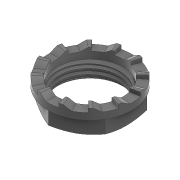
# Autodesk Inventor part: Switch Nut
Saved by Autodesk Inventor 2020 (Build 240168000, 168)
## iProperties
Created: 2019-11-13
Part Number: Switch Nut
Material: Generic
Document SubType Name: Modeling
Designer: amsmi
Density: 1 g/cm^3
Appearance: Default
Author: amsmi
Autodesk Inventor part; units mm, degrees
ref_plane "YZ Plane" through (0, 0, 0) normal (1, 0, 0) x (0, 1, 0)
ref_plane "XZ Plane" through (0, 0, 0) normal (0, 1, 0) x (-1, 0, 0)
sketch "Sketch1" plane through (0, 0, 0) normal (0, 1, 0) x (-1, 0, 0)
  circle A0 centre (0, 0) radius 5.842
  line L0 (6.985, 4.0328) -> (6.985, -4.0328)
  line L1 (6.985, -4.0328) -> (0, -8.0656)
  line L2 (0, -8.0656) -> (-6.985, -4.0328)
  line L3 (-6.985, -4.0328) -> (-6.985, 4.0328)
  line L4 (-6.985, 4.0328) -> (0, 8.0656)
  line L5 (0, 8.0656) -> (6.985, 4.0328)
  dimension "d0" = 11.684
  dimension "d1" = 13.97
  constraints: 12 end point, 2 coincident, 1 centre point, 1 vertical, 13 other
  measures "d0" diameter of A0
  measures "d1" distance between parallel lines of L3 L0
extrude "Extrusion1" add sketch "Sketch1" along normal blind 3.175
sketch "Sketch2" plane through (0, 3.175, 0) normal (0, 1, 0) x (1, 0, 0)
  circle A0 centre (0, 0) radius 8.128
  circle A1 centre (0, 0) radius 6.35
  dimension "d4" = 16.256
  dimension "d5" = 12.7
  constraints: 2 centre point, 2 coincident
  measures "d4" diameter of A0
  measures "d5" diameter of A1
extrude "Extrusion2" add sketch "Sketch2" along normal blind 2.159
chamfer "Chamfer1" distance 0.508 angle 45 2 edges at (5.842, 3.175, 0) (5.842, 0, 0)
sketch "Sketch3" plane through (0, 0, 0) normal (0, -1, 0) x (1, 0, 0)
  circle A0 centre (0, 0) radius 6.985
  line L0 (6.985, -4.0328) -> (0, -8.0656) projected
  constraints: 1 centre point, 1 coincident, 1 tangent
extrude "Extrusion3" cut sketch "Sketch3" against normal through all draft 60 keep common part
sketch "Sketch4" plane through (0, 0, 0) normal (0, 0, 1) x (1, 0, 0)
  line L0 (-1.905, 5.334) -> (-1.905, 4.445) construction
  line L1 (-1.905, 4.445) -> (0.381, 4.445) construction
  line L2 (0.381, 4.445) -> (1.905, 5.334) construction
  line L3 (1.905, 5.334) -> (-1.905, 5.334) construction
  line L4 (-6.35, 5.334) -> (6.35, 5.334) construction
  point P0 (0, 0)
  point P1 (0, 5.334)
  point P2 (0, 4.8895)
  point P3 (1.143, 4.8895)
  dimension "d29" = 3.81
  dimension "d30" = 2.286
  dimension "d31" = 0.889
  constraints: 8 end point, 2 horizontal, 2 midpoint, 2 vertical alignment, 1 horizontal alignment, 1 point on line, 1 vertical
  measures "d29" distance of L2.end L0.start
  measures "d30" distance of L0.end L1.end
  measures "d31" distance of L0.start L0.end
ref_plane "Work Plane1" through (0, 3.175, -8.128) normal (0, 0, 1) x (1, 0, 0)
sketch "Sketch5" plane through (0, 3.175, -8.128) normal (0, 0, 1) x (1, 0, 0)
  line L0 (-1.905, 1.27) -> (0.381, 1.27) projected
  line L1 (1.905, 2.159) -> (-1.905, 2.159) projected
  line L2 (0.381, 1.27) -> (1.905, 2.159) projected
  line L3 (-1.905, 2.159) -> (-1.905, 1.27) projected
  point P0 (0, -3.175)
loft "Loft1" cut profiles "Sketch5" section 2 point at (0, 4.8895, 0)
pattern_circular "Circular Pattern1" count 12 over 360 about axis through (0, 0, 0) along (0, 1, 0) of "Loft1"
thicken "Thicken2" operation cut thickness 0.127 both sides no extend neighbours no toward (0, -1, 0) faces at (0, 5.334, -6.9118)
sketch "Sketch6" plane through (0, 0, 0) normal (0, 0, 1) x (1, 0, 0)
  line L0 (-5.842, 2.667) -> (5.842, 2.667) construction
  line L1 (6.35, 3.175) -> (-6.35, 3.175) construction
  line L2 (-6.35, 0) -> (6.35, 0) construction
  line L3 (0, 3.175) -> (0, 0)
  line L4 (-5.842, 3.937) -> (-5.842, 3.175)
  line L5 (-5.842, 3.175) -> (-6.2819, 3.429)
  line L6 (-6.2819, 3.429) -> (-6.2819, 3.683)
  line L7 (-6.2819, 3.683) -> (-5.842, 3.937)
  dimension "d32" = 60
  dimension "d33" = 0.762
  dimension "d34" = 0.254
  dimension "d35" = 3.937
  constraints: 10 end point, 1 equal length, 1 midpoint, 1 parallel, 1 perpendicular, 1 point on line, 1 vertical, 1 vertical alignment
  measures "d32" angle of L5 L7
  measures "d33" distance of L4.start L4.end
  measures "d34" distance of L5.end L6.end
  measures "d35" distance from line of L2 L4.start
coil "Coil1" sketch "Sketch6" operation cut axis through (0, 3.175, 0) along (0, -1, 0) pitch 1.016 turns 3.875 hand right
equation "\"d34\" = 0.333333 * d33"
equation "\"d37\" = d35"
body "Solid1"
